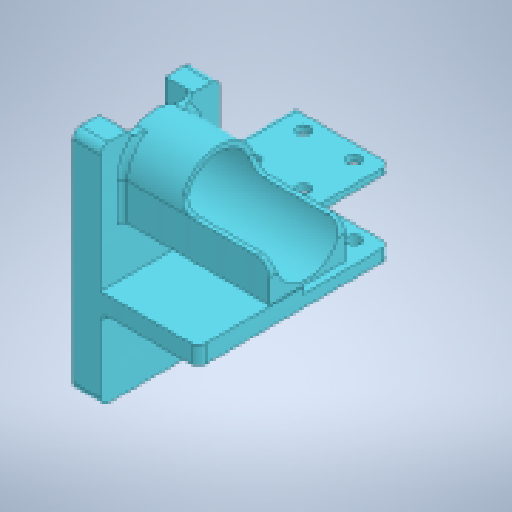
# Autodesk Inventor part: myMotorHolder
Saved by Autodesk Inventor 2024 (Build 280153000, 153)
## iProperties
Created: 2025-08-13
Part Number: myMotorHolder
Material: Типовые
Document SubType Name: Modeling
Designer: DELL
Density: 1 g/cm^3
Appearance: Серо-синий
Author: DELL
Autodesk Inventor part; units mm, degrees
ref_plane "YZ Plane" through (0, 0, 0) normal (1, 0, 0) x (0, 1, 0)
ref_plane "XZ Plane" through (0, 0, 0) normal (0, 1, 0) x (-1, 0, 0)
sketch "Эскиз1" plane through (0, 0, 0) normal (1, 0, 0) x (0, 1, 0)
  circle A0 centre (0, 0) radius 13
  circle A1 centre (0, 0) radius 15
  line L0 (0, -15) -> (-15, -15)
  line L1 (-15, -15) -> (-15, 15)
  line L2 (-15, 15) -> (0, 15)
  point P0 (-15, 0)
  dimension "d0" = 26
  dimension "d1" = 30
  constraints: 6 end point, 2 centre point, 2 coincident, 2 perpendicular, 2 point on circle, 2 tangent, 1 horizontal
  measures "d0" diameter of A0
  measures "d1" diameter of A1
extrude "Выдавливание1" add sketch "Эскиз1" along normal blind 60 contours A0 | A1 | A1 L1 L2 | L0 L1 A1
sketch "Эскиз2" plane through (60, 0, 0) normal (1, 0, 0) x (0, 0, 1)
  circle A0 centre (0, 0) radius 13
  dimension "d4" = 26
  constraints: 1 centre point, 1 coincident
  measures "d4" diameter of A0
extrude "Выдавливание2" cut sketch "Эскиз2" against normal blind 57
sketch "Эскиз3" plane through (0, 0, 0) normal (-1, 0, 0) x (0, 0, -1)
  circle A0 centre (0, 0) radius 3.6
  circle A1 centre (8.5, 0) radius 1.55
  circle A2 centre (-8.5, 0) radius 1.55
  line L0 (-8.5, 0) -> (8.5, 0) construction
  dimension "d7" = 7.2
  dimension "d8" = 3.1
  dimension "d9" = 3.1
  dimension "d10" = 17
  constraints: 3 centre point, 2 coincident, 2 end point, 1 horizontal, 1 midpoint
  measures "d7" diameter of A0
  measures "d8" diameter of A1
  measures "d9" diameter of A2
  measures "d10" distance of L0.start L0.end
extrude "Выдавливание3" cut sketch "Эскиз3" against normal blind 3
chamfer "Фаска1" distance 1.65 angle 45 2 edges at (0, 0, 10.05) (0, 0, -6.95)
sketch "Эскиз7" plane through (60, 0, 0) normal (1, 0, 0) x (0, 0, -1)
  arc A0 (15, 0) -> (-15, 0) centre (0, 0) ccw projected
  line L0 (-15, 0) -> (17, 0)
  line L1 (17, 0) -> (17, 16)
  line L2 (17, 16) -> (-15, 16)
  line L3 (-15, 16) -> (-15, 0)
  point P0 (15, 0)
  dimension "d25" = 32
  dimension "d26" = 16
  constraints: 8 end point, 2 parallel, 1 horizontal, 1 perpendicular
  measures "d25" distance of L2.end L1.end
  measures "d26" distance of L1.end L0.end
extrude "Выдавливание5" cut sketch "Эскиз7" against normal blind 35 contours L0 A0
fillet "Сопряжение1" radius 5 4 edges at (25, 0, 14) (25, 0, -14) (60, 0, -14) (60, 0, 14)
ref_plane "РабПлоскость5" through (0, -11, -14) normal (0, -1, 0) x (1, 0, 0)
sketch "Эскиз14" plane through (0, -15, -15) normal (0, 0, -1) x (-1, 0, 0)
  line L0 (-2, 3) -> (-62, 3)
  line L1 (-62, 3) -> (-62, 5.5)
  line L2 (-62, 5.5) -> (-2, 5.5)
  line L3 (0, 0) -> (-60, 0) projected
  line L4 (0, 0) -> (0, 15) projected
  line L5 (-2, 5.5) -> (-2, 3)
  point P0 (-2, 4.25)
  dimension "d66" = 60
  dimension "d67" = 2.5
  dimension "d68" = 3
  dimension "d96" = 60
  dimension "d141" = 2
  constraints: 8 end point, 1 horizontal, 1 midpoint, 1 parallel, 1 perpendicular
  measures "d66" distance of L1.end L2.end
  measures "d67" distance of L0.end L1.end
  measures "d68" distance between parallel lines of L3 L0
  measures "d96" distance of L0.start L0.end
  measures "d141" distance from line of L4 point (-2, 4.25)
extrude "Выдавливание11" add sketch "Эскиз14" along normal blind 37
sketch "Эскиз15" plane through (0, -15, -15) normal (0, -1, 0) x (1, 0, 0)
  line L0 (60, 30) -> (60, 0) projected
  line L1 (0, 0) -> (60, 0)
  line L2 (60, 0) -> (60, 30)
  line L3 (60, 30) -> (0, 30)
  line L4 (0, 30) -> (0, 0)
  dimension "d76" = 30
  constraints: 8 end point, 2 parallel, 1 horizontal, 1 perpendicular
  measures "d76" distance of L3.end L1.start
extrude "Выдавливание12" cut sketch "Эскиз15" against normal blind 0.5
sketch "Эскиз16" plane through (62, 2, 0) normal (1, 0, 0) x (0, 0, -1)
  line L0 (15, -11.5) -> (15, -14) projected
  line L1 (15, -14) -> (52, -14) projected
  line L2 (52, -11.5) -> (52, -14) projected
  line L3 (15, -11.5) -> (52, -11.5) projected
  point P0 (0, -2)
extrude "Выдавливание13" cut sketch "Эскиз16" against normal blind 21.5
fillet "Сопряжение4" radius 3 2 edges at (40.5, -10.75, -52) (21.25, -9.5, -15)
sketch "Эскиз17" plane through (0, -9.5, -18) normal (0, 1, 0) x (1, 0, 0)
  line L0 (2, 0) -> (2, 34) projected
  circle A0 centre (12, 28.5) radius 2.55 projected
  circle A1 centre (32, 28.5) radius 2.55 projected
  circle A2 centre (12, 8.5) radius 2.55 projected
  circle A3 centre (32, 8.5) radius 2.55 projected
  point P0 (0, -18)
extrude "Выдавливание14" cut sketch "Эскиз17" against normal blind 23
sketch "Эскиз18" plane through (0, 0, 0) normal (-1, 0, 0) x (0, 0, 1)
  line L0 (20.5, 15) -> (13, 15)
  line L1 (-23.5, 12) -> (-23.5, -71.1)
  line L2 (-20.5, -74.1) -> (20.5, -74.1)
  line L3 (23.5, -71.1) -> (23.5, 12)
  circle A0 centre (0, 0) radius 3.6 construction
  circle A1 centre (0, 0) radius 10 construction
  arc A2 (-13, 0) -> (13, 0) centre (0, 0) ccw
  line L4 (-13, 0) -> (-13, 15)
  circle A3 centre (0, 0) radius 13 construction
  line L5 (13, 0) -> (13, 15)
  line L6 (-13, 15) -> (-20.5, 15)
  line L7 (13, 15) -> (-13, 15) construction
  arc A4 (13, 0) -> (-13, 0) centre (0, 0) ccw construction
  circle A5 centre (0, -48.4) radius 18.65
  arc A6 (-23.5, -71.1) -> (-20.5, -74.1) centre (-20.5, -71.1) ccw
  arc A7 (20.5, -74.1) -> (23.5, -71.1) centre (20.5, -71.1) ccw
  arc A8 (-20.5, 15) -> (-23.5, 12) centre (-20.5, 12) ccw
  arc A9 (23.5, 12) -> (20.5, 15) centre (20.5, 12) ccw
  point P0 (-23.5, -74.1)
  point P1 (-23.5, 15)
  point P2 (23.5, -74.1)
  dimension "d85" = 47
  dimension "d86" = 89.1
  dimension "d87" = 23.5
  dimension "d88" = 15
  dimension "d89" = 20
  dimension "d90" = 26
  dimension "d91" = 37.3
  dimension "d92" = 48.4
  dimension "d93" = 3
  constraints: 16 end point, 13 point on circle, 9 perpendicular, 9 tangent, 8 centre point, 7 point on line, 4 parallel, 3 equal radius, 3 horizontal
  measures "d85" distance of point (23.5, -74.1) point (-23.5, -74.1)
  measures "d86" distance of point (-23.5, 15) point (-23.5, -74.1)
  measures "d87" distance from line of L3 A0.centre
  measures "d88" distance from line of L0 A0.centre
  measures "d89" diameter of A1
  measures "d90" diameter of A2
  measures "d91" diameter of A5
  measures "d92" distance of A5.centre A0.centre
  measures "d93" radius of A6
extrude "Выдавливание15" add sketch "Эскиз18" along normal blind 9
sketch "Эскиз19" plane through (0, 0, 0) normal (1, 0, 0) x (0, 0, -1)
  line L0 (-20.5, -74.1) -> (20.5, -74.1)
  line L1 (23.5, -71.1) -> (23.5, -16.5)
  line L2 (23.5, -16.5) -> (-23.5, -16.5)
  line L3 (-23.5, -16.5) -> (-23.5, -71.1)
  arc A0 (20.5, -74.1) -> (23.5, -71.1) centre (20.5, -71.1) ccw
  arc A1 (-23.5, -71.1) -> (-20.5, -74.1) centre (-20.5, -71.1) ccw
  point P0 (0, 0)
  point P1 (-23.5, -74.1)
  point P2 (23.5, -74.1)
  dimension "d98" = 47
  dimension "d102" = 3
  dimension "d118" = 57.6
  constraints: 8 end point, 4 point on circle, 4 point on line, 4 tangent, 2 centre point, 2 parallel, 1 equal radius, 1 horizontal, 1 perpendicular
  measures "d98" distance of L2.end L1.end
  measures "d102" radius of A0
  measures "d118" distance between parallel lines of L2 L0
extrude "Выдавливание16" add sketch "Эскиз19" along normal blind 2
sketch "Эскиз20" plane through (2, 0, 0) normal (1, 0, 0) x (0, 0, -1)
  circle A0 centre (0, -48.4) radius 18.65 construction
  circle A1 centre (0, -48.4) radius 2.5
  point P0 (0, 0)
  dimension "d103" = 5
  constraints: 1 centre point, 1 coincident
  measures "d103" diameter of A1
extrude "Выдавливание17" cut sketch "Эскиз20" against normal blind 5
sketch "Эскиз22" plane through (2, 0, 0) normal (1, 0, 0) x (0, 0, -1)
  circle A0 centre (0, -48.4) radius 8
  circle A1 centre (0, -48.4) radius 6.6
  circle A2 centre (0, -48.4) radius 2.5 projected
  point P0 (0, 0)
  dimension "d110" = 16
  dimension "d113" = 13.2
  constraints: 2 centre point, 2 coincident, 1 concentric
  measures "d110" diameter of A0
  measures "d113" diameter of A1
extrude "Выдавливание19" add sketch "Эскиз22" along normal blind 5 contours A0
sketch "Эскиз25" plane through (0, 0, 0) normal (1, 0, 0) x (0, 0, -1)
  line L0 (-23.5, -16.5) -> (23.5, -16.5) projected
  line L1 (-15, 0) -> (-15, -14.5) projected
  arc A0 (-13, 7.4833) -> (-15, 0) centre (0, 0) ccw projected
  line L2 (-13, 15) -> (-13, 7.4833) projected
  line L3 (-20.5, 15) -> (-13, 15) projected
  arc A1 (-20.5, 15) -> (-23.5, 12) centre (-20.5, 12) ccw projected
  line L4 (-23.5, -16.5) -> (-23.5, 12) projected
  line L5 (-23.5, -16.5) -> (23.5, -16.5) projected
  line L6 (23.5, 12) -> (23.5, -16.5) projected
  arc A2 (23.5, 12) -> (20.5, 15) centre (20.5, 12) ccw projected
  line L7 (13, 15) -> (20.5, 15) projected
  line L8 (13, 7.4833) -> (13, 15) projected
  arc A3 (15, 0) -> (13, 7.4833) centre (0, 0) ccw projected
  line L9 (-15, 0) -> (-15, -14.5) projected
  arc A4 (-13, 7.4833) -> (-15, 0) centre (0, 0) ccw projected
  line L10 (-13, 15) -> (-13, 7.4833) projected
  line L11 (-20.5, 15) -> (-13, 15) projected
  arc A5 (-20.5, 15) -> (-23.5, 12) centre (-20.5, 12) ccw projected
  line L12 (-23.5, -16.5) -> (-23.5, 12) projected
  line L13 (23.5, 12) -> (23.5, -16.5) projected
  arc A6 (23.5, 12) -> (20.5, 15) centre (20.5, 12) ccw projected
  line L14 (13, 15) -> (20.5, 15) projected
  line L15 (13, 7.4833) -> (13, 15) projected
  arc A7 (15, 0) -> (13, 7.4833) centre (0, 0) ccw projected
  line L16 (15, -14.5) -> (15, 0) projected
  line L17 (15, -14.5) -> (-15, -14.5) projected
  line L18 (15, -14.5) -> (15, 0) projected
  line L19 (15, -14.5) -> (-15, -14.5) projected
extrude "Выдавливание20" add sketch "Эскиз25" along normal blind 2
chamfer "Фаска4" distance 5 angle 20 1 edges at (2, -48.4, 8) measured on face at (2.5, -48.4, 8)
sketch "Эскиз26" plane through (2, 0, 0) normal (1, 0, 0) x (0, 0, -1)
  line L0 (-18, -74.1) -> (18, -74.1) construction
  line L1 (18, -74.1) -> (18, -34.5) construction
  line L2 (18, -34.5) -> (-18, -34.5) construction
  line L3 (-18, -34.5) -> (-18, -74.1) construction
  line L4 (18, -34.5) -> (-23.5, -34.5)
  line L5 (-23.5, -34.5) -> (-23.5, -37)
  line L6 (-23.5, -37) -> (18, -37)
  line L7 (18, -37) -> (18, -34.5)
  line L8 (-20.5, -74.1) -> (20.5, -74.1) construction
  line L9 (49, -12) -> (15, -12) projected
  line L10 (-23.5, -34.5) -> (18, -34.5)
  line L11 (18, -34.5) -> (18, -40.1)
  line L12 (18, -40.1) -> (-23.5, -40.1)
  line L13 (-23.5, -40.1) -> (-23.5, -34.5)
  line L14 (-15, -14.5) -> (15, -14.5) projected
  point P0 (0, 0)
  point P1 (0, -74.1)
  point P2 (-23.5, -35.75)
  dimension "d133" = 41.5
  dimension "d152" = 25
  dimension "d154" = 41.5
  dimension "d164" = 20
  constraints: 24 end point, 6 parallel, 3 horizontal, 3 midpoint, 3 perpendicular
  measures "d133" distance of L5.end L6.end
  measures "d152" distance between parallel lines of L9 L6
  measures "d154" distance of L11.end L12.end
  measures "d164" distance between parallel lines of L14 L4
extrude "Выдавливание21" add sketch "Эскиз26" along normal blind 38.5 contours L7 L6 L5 L4
fillet "Сопряжение5" radius 3 1 edges at (40.5, -35.75, 23.5)
sketch "Эскиз27" plane through (2, -37, -18) normal (0, -1, 0) x (1, 0, 0)
  arc A0 (35.5, -34) -> (38.5, -31) centre (35.5, -31) ccw
  line L0 (38.5, -31) -> (38.5, 0)
  line L1 (35.5, -34) -> (1.5, -34)
  line L2 (1.5, 0) -> (38.5, 0)
  line L3 (0, 41.5) -> (35.5, 41.5) projected
  line L4 (38.5, 0) -> (1.5, 0)
  line L5 (1.5, 0) -> (1.5, 41.5)
  line L6 (1.5, 41.5) -> (38.5, 41.5)
  line L7 (38.5, 41.5) -> (38.5, 0)
  line L8 (0, 38.5) -> (0, 41.5) projected
  line L9 (0, 41.5) -> (1.5, 41.5)
  line L10 (1.5, 41.5) -> (1.5, 0)
  line L11 (1.5, 0) -> (0, 0)
  line L12 (0, 0) -> (0, 41.5)
  line L13 (0, 0) -> (0, -34)
  line L14 (0, -34) -> (1.5, -34)
  circle A1 centre (30, -28.5) radius 2.55 projected
  circle A2 centre (10, -28.5) radius 2.55 projected
  circle A3 centre (10, -8.5) radius 2.55 projected
  circle A4 centre (30, -8.5) radius 2.55 projected
  point P0 (-2, 18)
  constraints: 26 end point, 4 parallel, 3 perpendicular, 2 centre point, 2 horizontal, 2 point on circle, 1 point on line, 1 vertical
extrude "Выдавливание22" add sketch "Эскиз27" along normal blind 2.5
fillet "Сопряжение6" radius 3 1 edges at (40.5, -38.25, 23.5)
fillet "Сопряжение9" radius 4 2 edges at (1, 7.4833, -13) (1, 7.4833, 13)
fillet "Сопряжение16" radius 2 7 edges at (2, 7.5721, -12.9485) (2, -8.6213, -15.8787) (2, -9.5, -20.75) (2, -9.5, -37.75) (2, -3.25, -15) (2, -7.25, 15) (2, 7.5721, 12.9485)
sketch "Эскиз29" plane through (2, 0, 0) normal (1, 0, 0) x (0, 0, -1)
  line L0 (-23.5, -39.5) -> (-23.5, -71.1) projected
  line L1 (-23.5, -39.5) -> (15, -39.5)
  line L2 (15, -39.5) -> (15, -41.6)
  line L3 (15, -41.6) -> (-23.5, -41.6)
  line L4 (-23.5, -41.6) -> (-23.5, -39.5)
  point P0 (0, 0)
  point P1 (-23.5, -37)
  dimension "d156" = 38.5
  dimension "d157" = 2.1
  constraints: 8 end point, 2 parallel, 1 horizontal, 1 perpendicular
  measures "d156" distance of L2.end L3.end
  measures "d157" distance of L1.end L2.end
extrude "Выдавливание23" add sketch "Эскиз29" along normal up to surface (38.5 mm away)
fillet "Сопряжение18" radius 3 1 edges at (40.5, -40.55, 23.5)
sketch "Эскиз30" plane through (2, -39.5, -18) normal (0, -1, 0) x (1, 0, 0)
  line L0 (38.5, 3) -> (0, 3) projected
  line L1 (0, -5.5) -> (0, 3) projected
  line L2 (0, -5.5) -> (0, -34) projected
  line L3 (0, -34) -> (35.5, -34) projected
  arc A0 (35.5, -34) -> (38.5, -31) centre (35.5, -31) ccw projected
  line L4 (38.5, -31) -> (38.5, 3) projected
  point P0 (-2, 18)
extrude "Выдавливание24" add sketch "Эскиз30" along normal up to surface (2.1 mm away)
fillet "Сопряжение19" radius 3 2 edges at (2, -41.6, 15.2922) (2, -41.6, -15.2922)
sketch "Эскиз31" plane through (2, -41.6, -52) normal (0, -1, 0) x (1, 0, 0)
  circle A0 centre (30, 25.5) radius 2.55 projected
  circle A1 centre (30, 5.5) radius 2.55 projected
  circle A2 centre (10, 5.5) radius 2.55 projected
  circle A3 centre (10, 25.5) radius 2.55 projected
  point P0 (-2, 52)
extrude "Выдавливание25" cut sketch "Эскиз31" against normal blind 2.5
